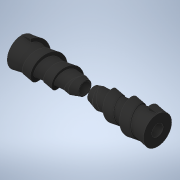
# Autodesk Inventor part: Dribblerschnecke2
Saved by Autodesk Inventor 2022 (Build 260153000, 153)
## iProperties
Part Number: Dribblerschnecke2
Material: Rubber, Silicone
Document SubType Name: Modeling
Designer: rYan
Mass: 61.7371 g
Surface Area: 150.716 cm^2
Volume: 49.3897 cm^3
Density: 1.25 g/cm^3
Appearance: Gummi - schwarz
Author: rYan
Autodesk Inventor part; units mm, degrees
ref_plane "YZ Plane" through (0, 0, 0) normal (1, 0, 0) x (0, 1, 0)
ref_plane "XZ Plane" through (0, 0, 0) normal (0, 1, 0) x (-1, 0, 0)
ref_plane "XY Plane" through (0, 0, 0) normal (0, 0, 1) x (1, 0, 0)
sketch "Skizze1" plane through (0, 0, 0) normal (1, 0, 0) x (0, 1, 0)
  circle A0 centre (0, 0) radius 3
  circle A1 centre (0, 0) radius 5.5
  dimension "d0" = 6
  dimension "d1" = 11
  constraints: 2 centre point, 2 coincident
  measures "d0" diameter of A0
  measures "d1" diameter of A1
extrude "Extrusion1" add sketch "Skizze1" along normal blind 36
sketch "Skizze3" plane through (0, 0, 0) normal (0, 1, 0) x (-1, 0, 0)
  line L0 (-36, 5.5) -> (-32, 5.5)
  line L1 (-32, 5.5) -> (-32.1763, 6.5)
  line L2 (-32.1763, 6.5) -> (-36, 5.6)
  line L3 (-36, 5.6) -> (-36, 5.5)
  line L4 (-36, 5.5) -> (-36, -5.5) construction
  line L5 (0, -5.5) -> (0, 5.5) construction
  point P0 (0, 0)
  dimension "d16" = 4
  dimension "d17" = 80
  dimension "d18" = 1
  dimension "d19" = 0.1
  constraints: 8 end point, 1 horizontal, 1 vertical
  measures "d16" distance of L0.start L0.end
  measures "d17" angle of L1 L0
  measures "d18" distance from line of L0 L1.end
  measures "d19" distance of L2.end L0.start
feature "Spirale1" [suppressed]
mirror "Spiegeln1" about plane through (0, 0, 0) normal (1, 0, 0) of "Extrusion1"
sketch "Sketch7" plane through (36, 0, 0) normal (1, 0, 0) x (0, 0, -1)
  line L0 (-10, -11) -> (10, -11)
  line L1 (10, -11) -> (10, 11)
  line L2 (10, 11) -> (-10, 11)
  line L3 (-10, 11) -> (-10, -11)
  line L4 (-10, -11) -> (10, 11) construction
  line L5 (10, -11) -> (-10, 11) construction
  point P0 (0, 0)
  constraints: 12 end point, 2 midpoint, 2 parallel, 1 horizontal, 1 perpendicular
extrude "Extrusion5" add sketch "Sketch7" along normal blind 10 and the other way blind 82 separate body
sketch "Sketch8" plane through (-46, 0, 0) normal (-1, 0, 0) x (0, 0, -1)
  circle A0 centre (0, 0) radius 3.5
  dimension "d34" = 7
  constraints: 1 centre point, 1 coincident
  measures "d34" diameter of A0
extrude "Extrusion6" add sketch "Sketch8" against normal up to surface (92 mm away) separate body
sketch "Sketch9" plane through (0, 0, 0) normal (0, 1, 0) x (-1, 0, 0)
  line L0 (36, 5.5) -> (-36, 5.5) projected
  line L1 (-36, 5.5) -> (-36, -5.5) projected
  line L2 (36, 5.5) -> (36, -5.5) projected
  line L3 (36, -5.5) -> (-36, -5.5) projected
  line L4 (36, -3) -> (36, 3) projected
  line L5 (-36, -3) -> (-36, 3) projected
  line L6 (36, 3) -> (-36, 3) projected
  line L7 (36, -3) -> (-36, -3) projected
  arc A0 (-36, 7.5) -> (36, 7.5) centre (0, 200) ccw
  line L8 (36, 7.5) -> (36, 5.5)
  line L9 (-36, 7.5) -> (-36, 5.5)
  line L10 (36, 0) -> (-36, 0) construction
  point P0 (0, 0)
  point P1 (22.8473, 5.5)
  point P2 (-22.8473, 5.5)
  dimension "d41" = 2
  dimension "d42" = 2
  dimension "d43" = 200
  constraints: 6 end point, 2 midpoint, 2 point on circle, 1 centre point, 1 parallel, 1 vertical
  measures "d41" distance of L0.end L9.start
  measures "d42" distance of L0.start L8.start
  measures "d43" distance of point (0, 0) A0.centre
revolve "Revolution1" add sketch "Sketch9" angle 360 about axis through (-36, 0, 0) along (1, 0, 0) bodies 1 contours L0 A0 L8 | L0 L9 A0
revolve "Revolution2" cut sketch "Sketch9" angle 360 about axis through (-36, 0, 0) along (1, 0, 0) bodies 1 contours A0 L0
sketch "Sketch10" plane through (0, 0, 0) normal (0, 1, 0) x (-1, 0, 0)
  arc A0 (-36, 7.5) -> (36, 7.5) centre (0, 200) ccw projected
  arc A1 (36, -7.5) -> (-36, -7.5) centre (0, -200) ccw projected
  line L0 (36, -7.5) -> (36, 7.5) projected
  line L1 (-36, 7.1) -> (-36, 7.7)
  line L2 (-36, 7.7) -> (-31.076, 8.4318)
  line L3 (-31.076, 8.4318) -> (-31.076, 6.2318)
  line L4 (-31.076, 6.2318) -> (-36, 7.1)
  line L5 (-36, -7.5) -> (-36, 7.5) projected
  line L6 (36, -3) -> (36, 3) projected
  line L7 (36, 0) -> (-36, 0) construction
  point P0 (0, 0)
  dimension "d47" = 0
  dimension "d48" = 80
  dimension "d49" = 5
  dimension "d50" = 2.2
  dimension "d51" = 0.6
  dimension "d61" = 80
  dimension "d62" = 7.1
  constraints: 10 end point, 2 midpoint, 1 vertical
  measures "d47" distance between parallel lines of L5 L1
  measures "d48" angle of L4 L3
  measures "d49" distance of L3.end L1.start
  measures "d50" distance of L3.end L2.end
  measures "d51" distance of L1.start L1.end
  measures "d61" angle of L5 L4
  measures "d62" vertical distance of point (0, 0) L1.start
coil "Coil2" sketch "Sketch10" operation add axis through (-36, 0, 0) along (-1, 0, 0) pitch 10 turns 3 hand right taper -6.9 bodies 1 contours L1 L2 L3 A0 | A0 L3 L4 L1
mirror "Mirror2" about plane through (0, 0, 0) normal (1, 0, 0) of "Coil2" bodies 1
sketch "Sketch11" plane through (0, 0, 0) normal (1, 0, 0) x (0, 1, 0)
  circle A0 centre (0, 0) radius 3 projected
extrude "Extrusion7" cut sketch "Sketch11" along normal mid plane 80 bodies 1
sketch "Sketch12" plane through (0, 0, 0) normal (1, 0, 0) x (0, 1, 0)
  circle A0 centre (0, 0) radius 3 projected
  circle A1 centre (0, 0) radius 7.5
  dimension "d65" = 15
  constraints: 1 centre point, 1 coincident
  measures "d65" diameter of A1
extrude "Extrusion8" cut sketch "Sketch12" along normal mid plane 5 bodies 1
sketch "Sketch13" plane through (0, 0, 0) normal (0, 1, 0) x (-1, 0, 0)
  line L0 (2.5, 3) -> (2.5, -3) projected
  line L1 (2.5, -4.1787) -> (2.5, 4.1787) projected
  line L2 (-2.5, 4.1787) -> (-2.5, -4.1787) projected
  line L3 (-2.5, -3) -> (-2.5, 3) projected
  arc A0 (2.5, 4.1787) -> (36, 7.5) centre (0, 200) ccw projected
  arc A1 (-36, 7.5) -> (-2.5, 4.1787) centre (0, 200) ccw projected
  line L4 (2.5, 0) -> (-2.5, 0) construction
  line L5 (-2.5, 4.5897) -> (-4.9522, 4.2253) projected
  line L6 (-2.5, 3.5) -> (-6, 4.5469)
  line L7 (2.5, 3.5) -> (6, 4.5469)
  line L8 (2.5, 4.5897) -> (4.9522, 4.2253) projected
  line L9 (-2.5, 4.1787) -> (-2.5, 4.5897) projected
  line L10 (2.5, 4.5897) -> (2.5, 4.1787) projected
  line L11 (-6, 4.5469) -> (-8.3387, 5.2095)
  line L12 (-8.3387, 5.2095) -> (-2.5, 5.2095)
  line L13 (-2.5, 5.2095) -> (-2.5, 4.5897)
  line L14 (6, 4.5469) -> (8.2153, 5.2095)
  line L15 (8.2153, 5.2095) -> (2.5, 5.2095)
  line L16 (2.5, 5.2095) -> (2.5, 4.5897)
  line L17 (8.2153, 5.2095) -> (2.5, 5.2095)
  line L18 (2.5, 5.2095) -> (2.5, 6.2095)
  line L19 (2.5, 6.2095) -> (8.2153, 6.2095)
  line L20 (8.2153, 6.2095) -> (8.2153, 5.2095)
  line L21 (-2.5, 5.2095) -> (-8.3387, 5.2095)
  line L22 (-8.3387, 5.2095) -> (-8.3387, 6.2095)
  line L23 (-8.3387, 6.2095) -> (-2.5, 6.2095)
  line L24 (-2.5, 6.2095) -> (-2.5, 5.2095)
  point P0 (0, 0)
  point P1 (-2.5, 2.6146)
  point P2 (6, 4.2546)
  point P3 (4.9522, 4.2253)
  point P4 (4.934, 4.228)
  point P5 (-4.934, 4.228)
  dimension "d68" = 3.5
  dimension "d69" = 3.5
  dimension "d71" = 1
  dimension "d72" = 0
  constraints: 34 end point, 4 parallel, 4 perpendicular, 3 horizontal, 2 collinear, 2 midpoint, 2 point on line, 2 other
  measures "d68" vertical distance of point (0, 0) L6.start
  measures "d69" vertical distance of point (0, 0) L7.start
  measures "d71" distance of L17.end L18.end
  measures "d72" distance between parallel lines of L12 L15
revolve "Revolution3" cut sketch "Sketch13" angle 360 about axis through (-2.5, 0, 0) along (1, 0, 0) bodies 1
equation "\"d41\" = d42"
body "Solid2"
body "Solid3"
